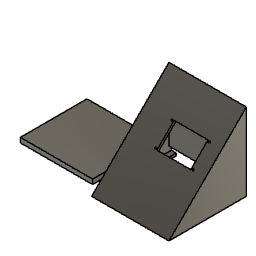
WeatherStation v1 (Autodesk Fusion 360 design; units mm, degrees)
Autodesk Fusion 360 part; units mm, degrees
note: some values were not read from the file. Set by a fixed rule: which sketch regions a step uses.
sketch "Sketch1" plane through (0, 0, 0) normal (0, 0, 1) x (1, 0, 0)
  line L0 (80, -80) -> (-80, -80)
  line L1 (-80, -80) -> (-80, 80)
  line L2 (-80, 80) -> (80, 80)
  line L3 (80, 80) -> (80, -80)
  line L4 (80, -80) -> (-80, 80) construction
  line L5 (-80, -80) -> (80, 80) construction
  dimension "d1" = 160
  dimension "d2" = 160
  constraint horizontal L0
  constraint perpendicular L0 L1
  constraint parallel L0 L2
  constraint parallel L1 L3
  constraint coincident L4 origin
  constraint coincident L5 origin
  measures "d1" distance of L1.end L2.end
  measures "d2" distance of L0.end L1.end
extrude "Extrude1" add sketch "Sketch1" along normal blind 160 makes body 1
sketch "Sketch2" plane through (80, 0, 0) normal (1, 0, 0) x (0, 1, 0)
  line L0 (-80, 0) -> (80, 0)
  line L1 (80, 0) -> (80, 160)
  line L2 (80, 160) -> (-80, 160)
  line L3 (-80, 160) -> (-80, 0)
  line L4 (-80, 0) -> (80, 160)
  line L5 (80, 160) -> (-80, 160)
  line L6 (-80, 160) -> (-80, 0)
  constraint coincident L0.start L3.end
  constraint coincident L1.end L2.start
  constraint coincident L2.end L3.start
extrude "Extrude2" cut sketch "Sketch2" against normal blind 160 contours L2 L3 L4 L5 L6 bodies 1
shell "Shell1" thickness 5 removed faces 1 at (26.6667, -26.6667, 0) on bodies 1
sketch "Sketch3" plane through (0, 80, 0) normal (0, 1, 0) x (-1, 0, 0)
  line L0 (-80, 0) -> (80, 0)
  line L1 (80, 0) -> (80, 160)
  line L2 (80, 160) -> (-80, 160)
  line L3 (-80, 160) -> (-80, 0)
  line L4 (-80, 0) -> (-80, 5)
  line L5 (80, 0) -> (80, 5)
  line L6 (-80, 0) -> (-65, 0)
  line L7 (80, 0) -> (65, 0)
  line L8 (65, 0) -> (65, 5)
  line L9 (65, 5) -> (75, 5)
  line L10 (75, 5) -> (75, 15)
  line L11 (75, 15) -> (-75, 15)
  line L12 (-75, 15) -> (-75, 5)
  line L13 (-75, 5) -> (-65, 5)
  line L14 (-65, 5) -> (-65, 0)
  line L15 (-65, 0) -> (65, 0)
  constraint coincident L0.start L3.end
  constraint coincident L3 L4.end
  constraint perpendicular L0 L4
  constraint coincident L0.end L1.start
  constraint coincident L1 L5.end
  constraint perpendicular L0 L5
  constraint coincident L0 L6.end
  constraint coincident L0 L7.end
  constraint perpendicular L7 L8
  constraint perpendicular L8 L9
  constraint perpendicular L9 L10
  constraint perpendicular L3 L11
  constraint perpendicular L11 L12
  constraint perpendicular L12 L13
  constraint perpendicular L6 L14
extrude "Extrude3" cut sketch "Sketch3" against normal blind 5 contours L0 L8 L9 L10 L11 L12 L13 L14 L15 bodies 1
sketch "Sketch4" plane through (0, 80, 0) normal (0, 1, 0) x (-1, 0, 0)
  line L0 (-65, 0) -> (-65, 5)
  line L1 (-65, 5) -> (-75, 5)
  line L2 (-75, 5) -> (-75, 15)
  line L3 (-75, 15) -> (75, 15)
  line L4 (75, 15) -> (75, 5)
  line L5 (75, 5) -> (65, 5)
  line L6 (65, 5) -> (65, 0)
  line L7 (65, 0) -> (80, 0)
  line L8 (80, 0) -> (80, 160)
  line L9 (80, 160) -> (-80, 160)
  line L10 (-80, 160) -> (-80, 0)
  line L11 (-80, 0) -> (-65, 0)
  line L12 (-75, 5) -> (-65, 5)
  line L13 (-65, 0) -> (-75, 0)
  line L14 (-75, 5) -> (-75, 0)
  line L15 (65, 5) -> (75, 5)
  line L16 (75, 0) -> (65, 0)
  line L17 (65, 5) -> (65, 0)
  line L18 (75, 5) -> (75, 0)
  constraint coincident L1.end L2.start
  constraint coincident L0.end L1.start
  constraint coincident L0.start L11.end
  constraint coincident L11 L13.end
  constraint perpendicular L0 L13
  constraint coincident L5.end L6.start
  constraint coincident L4.end L5.start
  constraint coincident L7 L16.start
  constraint coincident L6.end L7.start
  constraint perpendicular L6 L16
extrude "Extrude4" add sketch "Sketch4" against normal blind 155 contours L0 L1 L11 L12 L13 L14 | L5 L6 L7 L15 L16 L17 L18 bodies 1
sketch "Sketch5" plane through (0, -40, 40) normal (0, -0.707107, 0.707107) x (1, 0, 0)
  line L0 (80, -56.5685) -> (80, 169.7056)
  line L1 (80, 169.7056) -> (-80, 169.7056)
  line L2 (-80, 169.7056) -> (-80, -56.5685)
  line L3 (-80, -56.5685) -> (80, -56.5685)
  line L4 (80, 169.7056) -> (50, 169.7056)
  line L5 (50, 169.7056) -> (50, 100)
  line L6 (50, 100) -> (80, 100)
  line L7 (50, 169.7056) -> (-20, 169.7056)
  line L8 (-20, 100) -> (-20, 169.7056)
  line L9 (-20, 100) -> (50, 100)
  line L10 (-20, 100) -> (-80, 100)
  line L11 (-20, 100) -> (50, 100)
  line L12 (50, 100) -> (50, 49.67)
  line L13 (50, 49.67) -> (-20, 49.67)
  line L14 (-20, 49.67) -> (-20, 100)
  line L15 (-20, 100) -> (50, 100)
  line L16 (50, 100) -> (50, 98.3)
  line L17 (50, 98.3) -> (53.8, 98.3)
  circle A0 centre (53.8, 98.3) radius 1.78
  line L18 (-20, 100) -> (-23.8, 100)
  line L19 (-20, 100) -> (-20, 98.3)
  line L20 (-23.8, 100) -> (-23.8, 98.3)
  line L21 (-23.8, 98.3) -> (-20, 98.3)
  circle A1 centre (-23.8, 98.3) radius 1.78
  line L22 (-20, 49.67) -> (-20, 51.35)
  line L23 (-20, 49.67) -> (-23.8, 49.67)
  line L24 (-23.8, 49.67) -> (-23.8, 51.35)
  line L25 (-23.8, 51.35) -> (-20, 51.35)
  circle A2 centre (-23.8, 51.35) radius 1.78
  line L26 (50, 49.67) -> (53.8, 49.67)
  line L27 (50, 49.67) -> (50, 51.35)
  line L28 (50, 51.35) -> (53.8, 51.35)
  line L29 (53.8, 51.35) -> (53.8, 49.67)
  circle A3 centre (53.8, 51.35) radius 1.78
  dimension "d12" = 50.33
  dimension "d13" = 1.7
  dimension "d14" = 3.8
  dimension "d15" = 3.56
  dimension "d16" = 3.8
  dimension "d17" = 1.7
  dimension "d18" = 1.7
  dimension "d19" = 3.8
  dimension "d20" = 3.56
  dimension "d21" = 1.68
  dimension "d22" = 3.8
  dimension "d23" = 1.68
  dimension "d24" = 3.56
  dimension "d25" = 3.8
  dimension "d26" = 1.68
  dimension "d27" = 3.8
  dimension "d28" = 1.68
  dimension "d29" = 3.56
  constraint coincident L0.end L1.start
  constraint coincident L1 L4.end
  constraint perpendicular L4 L5
  constraint coincident L0 L6.end
  constraint perpendicular L0 L6
  constraint coincident L1 L7.end
  constraint perpendicular L7 L8
  constraint perpendicular L5 L9
  constraint coincident L2 L10.end
  constraint perpendicular L2 L10
  constraint perpendicular L11 L12
  constraint parallel L11 L13
  constraint parallel L12 L14
  constraint perpendicular L6 L16
  constraint perpendicular L12 L17
  constraint coincident L17.end A0.centre
  constraint perpendicular L14 L18
  constraint perpendicular L15 L19
  constraint perpendicular L10 L20
  constraint perpendicular L20 L21
  constraint coincident L20.end L21.start
  constraint perpendicular L13 L22
  constraint perpendicular L22 L23
  constraint perpendicular L23 L24
  constraint coincident L24.end L25.start
  constraint perpendicular L12 L26
  constraint perpendicular L13 L27
  constraint perpendicular L12 L28
  constraint perpendicular L26 L29
  constraint coincident L28.end L29.start
  measures "d12" distance of L8.start L13.end
  measures "d13" distance of L5.end L16.end
  measures "d14" distance of L16.end L17.end
  measures "d15" diameter of A0
  measures "d16" distance of L8.start L18.end
  measures "d17" distance of L8.start L19.end
  measures "d18" distance of L18.end L20.end
  measures "d19" distance of L20.end L19.end
  measures "d20" diameter of A1
  measures "d21" distance of L13.end L22.end
  measures "d22" distance of L13.end L23.end
  measures "d23" distance of L23.end L24.end
  measures "d24" diameter of A2
  measures "d25" distance of L12.end L26.end
  measures "d26" distance of L12.end L27.end
  measures "d27" distance of L27.end L28.end
  measures "d28" distance of L28.end L26.end
  measures "d29" diameter of A3
extrude "Extrude5" cut sketch "Sketch5" against normal blind 5 contours L6 A0 | L6 A0 | L10 L18 A1 | L10 L20 L21 A1 | L9 L11 L12 L13 L14 L15 L16 L19 L22 L27 | L10 L18 L20 L21 A1 | L26 L28 L29 A3 | L26 L28 L29 A3 | L23 L24 L25 A2 | L23 L24 L25 A2 bodies 1
sketch "Sketch6" plane through (0, 0, 0) normal (0, 0, 1) x (1, 0, 0)
  line L0 (-100, 80) -> (-249.6, 80)
  line L1 (-249.6, 80) -> (-249.6, -57.9289)
  line L2 (-249.6, -57.9289) -> (-100, -57.9289)
  line L3 (-100, -57.9289) -> (-100, 80)
  dimension "d32" = 149.6
  dimension "d33" = 137.9289
  constraint horizontal L0
  constraint vertical L1
  constraint horizontal L2
  constraint vertical L3
  measures "d32" distance of L0.start L0.end
  measures "d33" distance of L0.start L2.end
extrude "Extrude6" add sketch "Sketch6" along normal blind 9.8 separate body makes body 2
equation "d15 = 1.78 mm * 2"
equation "d20 = ( 1.78 * 2 ) * 1 mm"
equation "d33 = 145 mm - 7.07107 mm"
